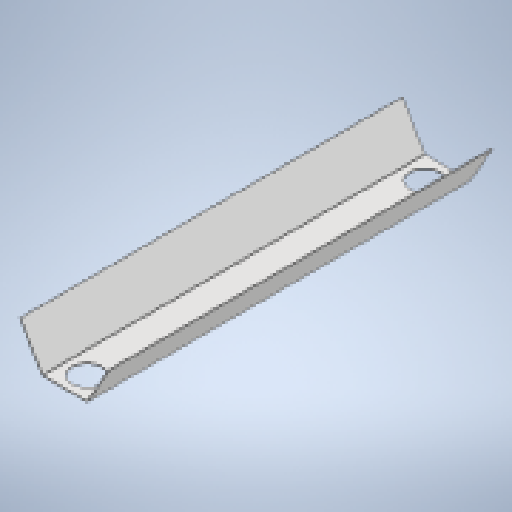
# Autodesk Inventor part: DSB 122 hex side 1
Saved by Autodesk Inventor 2025 (Build 290162010, 162A)
## iProperties
Created: 2024-12-09
Part Number: DSB 122 hex side 1
Material: Generic
Document SubType Name: Sheet Metal
Designer: user
Mass: 562.517 g
Surface Area: 5683.88 cm^2
Volume: 562.517 cm^3
Density: 1 g/cm^3
Sheet Metal Rule: Default
Sheet Metal Width: 318,794 mm
Sheet Metal Length: 910,000 mm
Sheet Metal Area: 290102,771 mm^2
Appearance: Default
Flat Pattern Width: 31.8794 cm
Flat Pattern Length: 91 cm
Flat Pattern Area: 2901.03 cm^2
Octaeder_side: 55.919 mm
Octaeder_flange_lenth: 72.500 mm
Author: user
Autodesk Inventor part; units mm, degrees
ref_plane "YZ Plane" through (0, 0, 0) normal (1, 0, 0) x (0, 1, 0)
ref_plane "XZ Plane" through (0, 0, 0) normal (0, 1, 0) x (-1, 0, 0)
ref_plane "XY Plane" through (0, 0, 0) normal (0, 0, 1) x (1, 0, 0)
sketch "Sketch9" plane through (0, 0, 0) normal (0, 0, 1) x (1, 0, 0)
  line L0 (-54, 0) -> (54, 0)
  line L1 (54, 0) -> (54, -910)
  line L2 (54, -910) -> (-54, -910)
  line L3 (-54, -910) -> (-54, 0)
  point P0 (0, 0)
  point P1 (0, 0)
  dimension "d49" = 108
  dimension "d50" = 910
  measures "d49" distance of L1.end L2.end
  measures "d50" distance of L0.end L1.end
extrude "Plate4" add sketch "Sketch9" along normal blind 2
sketch "Sketch10" plane through (52.2679, 0, 1) normal (0.8660254, 0, -0.5) x (0, 1, 0)
  line L0 (-910, 0) -> (0, 0)
  line L1 (0, 0) -> (0, 107)
  line L2 (0, 107) -> (-910, 107)
  line L3 (-910, 107) -> (-910, 0)
  constraints: 6 end point, 1 horizontal, 1 perpendicular, 1 vertical
edge flange "Flange2" height 107 angle 60 thickness 2 bend radius 2 thickness toward (0.8660254, 0, -0.5) relief tear relief width 2 relief depth 1 corner gap 2 corner form 0 edges at (54, -455, 2) (-54, -455, 2) wall of the first edge with corners at (52.2679, -910, 1) (52.2679, 0, 1) (105.7679, 0, 93.6647) (105.7679, -910, 93.6647)
bend "Bend2"
corner "Corner2"
sketch "Sketch11" plane through (0, 0, 2) normal (0, 0, 1) x (1, 0, 0)
  circle A0 centre (0, -53) radius 36
  circle A1 centre (0, -857) radius 36
  line L0 (-51.6906, 0) -> (51.6906, 0) projected
  line L1 (-51.6906, -910) -> (51.6906, -910) projected
  line L2 (0, 0) -> (0, -17)
  line L3 (0, -910) -> (0, -893)
  point P0 (0, 0)
  dimension "d62" = 72
  dimension "d68" = 17
  dimension "d69" = 804
  constraints: 4 end point, 4 vertical alignment, 3 midpoint, 2 vertical, 1 collinear, 4 other
  measures "d68" distance of L2.start L2.end
  measures "d69" distance of point (0, -857) point (0, -53)
extrude "Cut3" cut sketch "Sketch11" against normal blind 2
equation "\"d65\" = Thickness"
equation "\"d51\" = Thickness"
equation "\"d52\" = BendReliefWidth"
equation "\"d53\" = BendReliefDepth"
equation "\"d54\" = MinimumRemnant"
equation "\"d55\" = TransitionRadius"
equation "\"d58\" = BendRadius"
equation "\"d59\" = CornerReliefSize"
equation "\"d60\" = GapSize"
equation "\"d61\" = JacobiRadiusSize"
equation "\"BendRadius\" = Thickness"
equation "\"BendReliefWidth\" = Thickness"
equation "\"BendReliefDepth\" = 0.5 * Thickness"
equation "\"CornerReliefSize\" = 4 * Thickness"
equation "\"MinimumRemnant\" = 2 * Thickness"
equation "\"TransitionRadius\" = BendRadius"
equation "\"JacobiRadiusSize\" = BendRadius"
equation "\"GapSize\" = Thickness"
equation "\"Octaeder_side\" = d41"
equation "\"Octaeder_flange_lenth\" = d42"
equation "\"Thickness\" = 2"
equation "\"d41\" = 55.918831"
equation "\"d42\" = 72.5"
body "Solid3"
